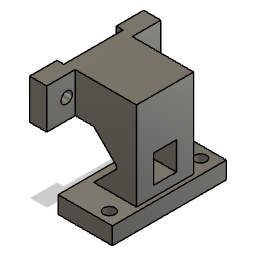
支架 v1 (Autodesk Fusion 360 design; units mm, degrees)
Autodesk Fusion 360 part; units mm, degrees
sketch "草图1" plane through (0, 0, 0) normal (1, 0, 0) x (0, 0, -1)
  line L0 (0, 15) -> (0, -11)
  line L1 (0, 0) -> (0, 3.5)
  line L2 (0, 3.5) -> (-10, 3.5)
  line L3 (-10, 3.5) -> (10, 3.5)
  line L4 (10, 3.5) -> (10, -3.5)
  line L5 (10, -3.5) -> (-10, -3.5)
  line L6 (-10, -3.5) -> (-10, 3.5)
  circle A0 centre (-6.5, 0) radius 3.5
  circle A1 centre (6.5, 0) radius 3.5
  circle A2 centre (-6.5, 0) radius 1
  circle A3 centre (6.5, 0) radius 1
  dimension "d1" = 3.5
  dimension "d2" = 10
  dimension "d3" = 20
  dimension "d4" = 7
  dimension "d5" = 7
  dimension "d6" = 2
  constraint vertical L0
  constraint coincident L1.start origin
  constraint parallel L0 L1
  constraint perpendicular L1 L2
  constraint horizontal L3
  constraint vertical L4
  constraint horizontal L5
  constraint vertical L6
  constraint tangent L6 A0
  constraint tangent L3 A0
  constraint symmetric L0 A0 A1
  constraint concentric A0 A2
  constraint symmetric L0 A2 A3
  measures "d1" distance of L1.start L1.end
  measures "d2" distance of L1.end L2.end
  measures "d3" distance of L2.end L3.end
  measures "d4" distance of L2.end L5.end
  measures "d5" diameter of A0
  measures "d6" diameter of A2
extrude "拉伸1" add sketch "草图1" along normal blind 3
sketch "草图2" plane through (0, 0, 0) normal (-1, 0, 0) x (0, 0, 1)
  circle A0 centre (6.5, 0) radius 1
  circle A1 centre (-6.5, 0) radius 1
  line L0 (-10, -3.5) -> (10, -3.5)
  line L1 (10, -3.5) -> (10, 3.5)
  line L2 (10, 3.5) -> (-10, 3.5)
  line L3 (-10, 3.5) -> (-10, -3.5)
  line L4 (-5.1992, 3.5) -> (-5.1992, -3.6)
  line L5 (0, 12) -> (0, -5)
  line L6 (5.1992, 3.5) -> (5.1992, -3.6)
  line L7 (-5.1992, 3.5) -> (5.1992, 3.5)
  line L8 (-5.1992, -3.5) -> (5.1992, -3.5)
  point P0 (0, -5)
  constraint coincident L2 L4.start
  constraint perpendicular L0 L4
  constraint perpendicular L0 L5
  constraint midpoint L2 L5
  constraint symmetric L4.start L5 L6.start
  constraint symmetric L4.end L5 L6.end
  constraint symmetric P0 L5 L5.end
  constraint coincident L4 L8.start
  constraint coincident L0 L8.start
  constraint coincident L6 L8.end
  constraint coincident L0 L8.end
  constraint perpendicular L6 L8
extrude "拉伸2" cut sketch "草图2" against normal blind 1.2 contours L0 L2 L4 L5 L7 L8 | L0 L2 L5 L6 L7 L8
sketch "草图3" plane through (3, 0, 0) normal (1, 0, 0) x (0, 0, -1)
  circle A0 centre (-6.5, 0) radius 1
  circle A1 centre (6.5, 0) radius 1
  line L0 (-10, -3.5) -> (10, -3.5)
  line L1 (10, -3.5) -> (10, 3.5)
  line L2 (10, 3.5) -> (-10, 3.5)
  line L3 (-10, 3.5) -> (-10, -3.5)
  line L4 (-5.0058, 3.5) -> (-5.0058, -3.5)
  line L5 (0, 10.9) -> (0, -3.9)
  line L6 (5.0058, 3.5) -> (5.0058, -3.5)
  point P0 (0, -3.9)
  constraint coincident L2 L4.start
  constraint coincident L0 L4.end
  constraint perpendicular L0 L4
  constraint perpendicular L0 L5
  constraint midpoint L2 L5
  constraint symmetric L4.start L5 L6.start
  constraint symmetric L4.end L5 L6.end
  constraint symmetric P0 L5 L5.end
extrude "拉伸3" add sketch "草图3" along normal blind 10.75 contours L0 L2 L4 L5 | L0 L2 L5 L6
sketch "草图4" plane through (0, -3.5, 0) normal (0, -1, 0) x (1, 0, 0)
  line L0 (1.2, -5.1992) -> (0, -5.1992)
  line L1 (0, -5.1992) -> (0, -10)
  line L2 (0, -10) -> (3, -10)
  line L3 (3, -10) -> (3, -5.0058)
  line L4 (3, -5.0058) -> (13.75, -5.0058)
  line L5 (13.75, -5.0058) -> (13.75, 5.0058)
  line L6 (13.75, 5.0058) -> (3, 5.0058)
  line L7 (3, 5.0058) -> (3, 10)
  line L8 (3, 10) -> (0, 10)
  line L9 (0, 10) -> (0, 5.1992)
  line L10 (0, 5.1992) -> (1.2, 5.1992)
  line L11 (1.2, 5.1992) -> (1.2, -5.1992)
  line L12 (13.75, 5.0058) -> (10.25, 5.0058)
  line L13 (10.25, 5.0058) -> (10.25, -5.0058)
  line L14 (10.25, -5.0058) -> (13.75, -5.0058)
  line L15 (13.75, -5.0058) -> (13.75, 5.0058)
  line L16 (10.25, -5.0058) -> (10.25, 5.0058)
  line L17 (10.25, 5.0058) -> (13.75, 5.0058)
  dimension "d13" = 3.5
  constraint horizontal L12
  constraint vertical L13
  constraint horizontal L14
  constraint vertical L15
  constraint coincident L5.end L6.start
  measures "d13" distance of L5.end L12.end
extrude "拉伸4" add sketch "草图4" along normal blind 8.5 contours L4 L5 L6 L12 L13 L14 L15 L16 L17
sketch "草图5" plane through (0, -12, 0) normal (0, -1, 0) x (1, 0, 0)
  line L0 (10.25, -5.0058) -> (13.75, -5.0058)
  line L1 (13.75, -5.0058) -> (13.75, 5.0058)
  line L2 (13.75, 5.0058) -> (10.25, 5.0058)
  line L3 (10.25, 5.0058) -> (10.25, -5.0058)
  line L4 (10.25, 5.0058) -> (13.75, 5.0058)
  line L5 (13.75, 5.0058) -> (13.75, 8.5058)
  line L6 (13.75, 8.5058) -> (10.25, 8.5058)
  line L7 (10.25, 8.5058) -> (10.25, 5.0058)
  line L8 (-5, 0) -> (20, 0)
  line L9 (13.75, -8.5058) -> (10.25, -8.5058)
  line L10 (10.25, -8.5058) -> (10.25, -5.0058)
  line L11 (10.25, -5.0058) -> (13.75, -5.0058)
  line L12 (13.75, -5.0058) -> (13.75, -8.5058)
  line L13 (13.75, 8.5058) -> (13.75, -8.5058)
  line L14 (13.75, 8.5058) -> (14.5, 8.5058)
  line L15 (14.5, 8.5058) -> (14.5, -8.5062)
  line L16 (14.5, -8.5062) -> (13.75, -8.5062)
  line L17 (13.75, -8.5062) -> (13.75, 8.5058)
  line L18 (12, 28.0115) -> (12, -11)
  line L19 (10.25, 8.5058) -> (9.5, 8.5058)
  line L20 (9.5, 8.5058) -> (9.5, -8.5062)
  line L21 (9.5, -8.5062) -> (10.25, -8.5062)
  line L22 (10.25, -8.5062) -> (10.25, 8.5058)
  dimension "d16" = 3.5
  dimension "d17" = 3.5
  dimension "d19" = 17.0115
  dimension "d20" = 0.75
  dimension "d21" = 17.012
  dimension "d22" = 0.75
  dimension "d23" = 17.012
  constraint horizontal L4
  constraint vertical L5
  constraint horizontal L6
  constraint vertical L7
  constraint coincident L2.end L3.start
  constraint horizontal L8
  constraint symmetric L2.end L8 L0.start
  constraint symmetric L1.end L8 L0.end
  constraint symmetric L6.end L8 L9.end
  constraint perpendicular L9 L13
  constraint horizontal L14
  constraint vertical L15
  constraint horizontal L16
  constraint vertical L17
  constraint perpendicular L9 L18
  constraint midpoint L6 L18
  constraint horizontal L19
  constraint vertical L20
  constraint horizontal L21
  constraint vertical L22
  measures "d16" distance of L2.end L1.end
  measures "d17" distance of L2.end L6.end
  measures "d19" distance of L5.end L9.start
  measures "d20" distance of L5.end L14.end
  measures "d21" distance of L5.end L16.end
  measures "d22" distance of L6.end L19.end
  measures "d23" distance of L6.end L21.end
extrude "拉伸5" add sketch "草图5" along normal blind 3
sketch "草图6" plane through (0, -15, 0) normal (0, -1, 0) x (1, 0, 0)
  line L0 (9.5, 8.5058) -> (9.5, -8.5062)
  line L1 (9.5, -8.5062) -> (10.25, -8.5062)
  line L2 (10.25, -8.5062) -> (10.25, -8.5058)
  line L3 (10.25, -8.5058) -> (13.75, -8.5058)
  line L4 (13.75, -8.5058) -> (13.75, -8.5062)
  line L5 (13.75, -8.5062) -> (14.5, -8.5062)
  line L6 (14.5, -8.5062) -> (14.5, 8.5058)
  line L7 (14.5, 8.5058) -> (9.5, 8.5058)
  line L8 (19.5, 0) -> (-2, 0)
  line L9 (14.5, -0.0002) -> (14.5, -10.0002)
  line L10 (14.5, -0.0002) -> (14.5, 9.9998)
  line L11 (9.5, 8.5058) -> (9.5, 14.5)
  line L12 (14.5, 9.9998) -> (9.5, 9.9998)
  line L13 (9.5, -8.5062) -> (9.5, -12.5)
  line L14 (14.5, -10.0002) -> (9.5, -10.0002)
  dimension "d26" = 10
  dimension "d27" = 10
  constraint perpendicular L0 L8
  constraint midpoint L6 L9.start
  constraint perpendicular L8 L9
  constraint perpendicular L7 L10
  constraint coincident L0.start L7.end
  constraint perpendicular L7 L11
  constraint coincident L11 L12.end
  constraint perpendicular L11 L12
  constraint coincident L0.end L1.start
  constraint perpendicular L1 L13
  constraint coincident L13 L14.end
  constraint perpendicular L13 L14
  measures "d26" distance of L9.start L9.end
  measures "d27" distance of L9.start L10.end
extrude "拉伸6" add sketch "草图6" against normal blind 3 contours L7 L10 L11 L12 | L1 L3 L5 L9 L13 L14
sketch "草图7" plane through (0, -15, 0) normal (0, -1, 0) x (1, 0, 0)
  line L0 (9.5, 9.9998) -> (9.5, -10.0002)
  line L1 (9.5, -10.0002) -> (14.5, -10.0002)
  line L2 (14.5, -10.0002) -> (14.5, 9.9998)
  line L3 (14.5, 9.9998) -> (9.5, 9.9998)
  line L4 (12, 37.9995) -> (12, -18)
  line L5 (14.5, 9.9998) -> (14.5, 7.9998)
  line L6 (14.5, 7.9998) -> (12, 7.9998)
  line L7 (19, 0) -> (-4.5239, -0.0002)
  circle A0 centre (12, 7.9998) radius 1
  circle A1 centre (12.0002, -7.9999) radius 1
  dimension "d30" = 2
  dimension "d31" = 2
  constraint perpendicular L1 L4
  constraint midpoint L3 L4
  constraint coincident L2.end L3.start
  constraint perpendicular L3 L5
  constraint coincident L4 L6.end
  constraint perpendicular L4 L6
  constraint coincident L6.end A0.centre
  constraint symmetric L7 A0 A1
  measures "d30" distance of L2.end L5.end
  measures "d31" diameter of A0
extrude "拉伸7" cut sketch "草图7" against normal blind 3 contours L4 L6 A0 | L4 A0 | L4 L6 A0 | L4 A1 | L4 A1
sketch "草图8" plane through (13.75, 0, 0) normal (1, 0, 0) x (0, 0, -1)
  line L0 (-5.0058, 3.5) -> (-5.0058, -12)
  line L1 (-5.0058, -12) -> (5.0058, -12)
  line L2 (5.0058, -12) -> (5.0058, 3.5)
  line L3 (5.0058, 3.5) -> (-5.0058, 3.5)
  line L4 (9.4841, 8.7498) -> (9.4841, -23.2502)
  line L5 (9.4841, -7.2502) -> (12.4841, -7.2502)
  line L6 (12.4841, -7.2502) -> (6.4841, -7.2502)
  line L7 (6.4841, -7.2502) -> (6.4841, -11.2502)
  line L8 (6.4841, -11.2502) -> (12.4841, -11.2502)
  line L9 (12.4841, -11.2502) -> (12.4841, -7.2502)
  line L10 (0, 25.2099) -> (0, -18.2099)
  line L11 (0, -6.5) -> (2, -6.5)
  line L12 (2, -6.5) -> (2, -9)
  line L13 (2, -9) -> (0, -9)
  line L14 (-2, -6.5) -> (-2, -9)
  line L15 (0, -6.5) -> (-2, -6.5)
  line L16 (-2, -9) -> (0, -9)
  line L17 (-2, -6.5) -> (-2, -5.3)
  line L18 (2, -6.5) -> (2, -5.3)
  line L19 (2, -9) -> (2, -10.2)
  line L20 (-2, -9) -> (-2, -10.2)
  line L21 (-2, -10.2) -> (2, -10.2)
  line L22 (2, -5.3) -> (1.9, -5.3)
  line L23 (1.9, -5.3) -> (-2, -5.3)
  dimension "d35" = 3
  dimension "d36" = 6
  dimension "d37" = 4
  dimension "d46" = 2
  dimension "d47" = 1.2
  dimension "d48" = 1.2
  constraint perpendicular L1 L4
  constraint midpoint L4 L5.start
  constraint perpendicular L4 L5
  constraint horizontal L6
  constraint vertical L7
  constraint horizontal L8
  constraint vertical L9
  constraint parallel L4 L10
  constraint midpoint L3 L10
  constraint coincident L10 L11.start
  constraint perpendicular L10 L11
  constraint perpendicular L11 L12
  constraint coincident L10 L13.end
  constraint perpendicular L10 L13
  constraint symmetric L10 L11.start L15.start
  constraint symmetric L10 L11.end L14.start
  constraint symmetric L10 L12.end L14.end
  constraint symmetric L10 L13.end L16.end
  constraint perpendicular L15 L17
  constraint perpendicular L11 L18
  constraint perpendicular L13 L19
  constraint perpendicular L16 L20
  constraint perpendicular L18 L22
  measures "d35" distance of L5.start L5.end
  measures "d36" distance of L5.end L6.end
  measures "d37" distance of L5.end L8.end
  measures "d46" distance of L11.start L11.end
  measures "d47" distance of L11.end L18.end
  measures "d48" distance of L12.end L19.end
extrude "拉伸11" cut sketch "草图8" against normal blind 3.5 contours L10 L11 L18 L22 L23 | L10 L15 L17 L23 | L10 L16 L20 L21 | L10 L13 L19 L21 | L10 L11 L12 L13 | L10 L14 L15 L16
extrude "拉伸9" cut sketch "草图8" against normal blind 3.5 contours L4 L5 L6 L8 L9 | L4 L6 L7 L8
extrude "拉伸8" cut sketch "草图8" against normal blind 3.5 contours L4 L5 L6 L8 L9 | L4 L6 L7 L8
sketch "草图9" plane through (0, -15, 0) normal (0, -1, 0) x (1, 0, 0)
  circle A0 centre (12, 7.9998) radius 1
  circle A1 centre (12.0002, -7.9999) radius 1
  line L0 (9.5, 9.9998) -> (9.5, -10.0002)
  line L1 (9.5, -10.0002) -> (14.5, -10.0002)
  line L2 (14.5, -10.0002) -> (14.5, 9.9998)
  line L3 (14.5, 9.9998) -> (9.5, 9.9998)
  line L4 (9.5, 9.9998) -> (9.5, -10.0002)
  line L5 (9.5, 9.9998) -> (5, 9.9998)
  line L6 (5, 9.9998) -> (5, -10)
  line L7 (5, -10) -> (9.5, -10.0002)
  constraint coincident L0.start L3.end
  constraint coincident L0.end L1.start
  constraint perpendicular L0 L5
  constraint perpendicular L5 L6
extrude "拉伸10" add sketch "草图9" against normal blind 3 contours L0 L4 L5 L6 L7
chamfer "倒角1" distance 4 angle 45 1 edges at (10.25, -3.5, 0)
chamfer "倒角2" distance 4 angle 45 1 edges at (10.25, -12, 0)
